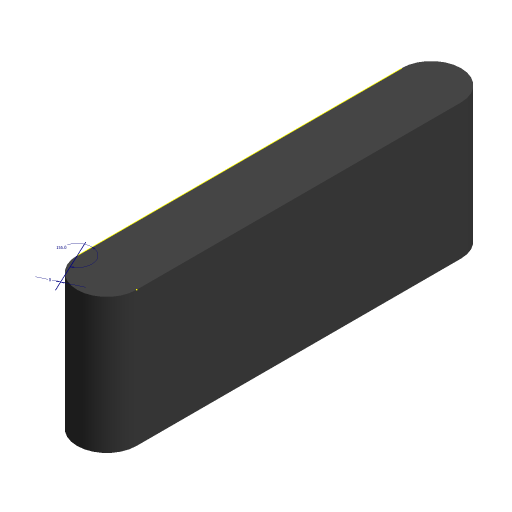
# Autodesk Inventor part: Camera retention
Saved by Autodesk Inventor 2024 (Build 280153000, 153)
## iProperties
Part Number: Camera retention
Material: Generic
Document SubType Name: Modeling
Designer: Jamie
Appearance: Default
Author: Jamie
Autodesk Inventor part; units mm, degrees
ref_plane "YZ Plane" through (0, 0, 0) normal (1, 0, 0) x (0, 1, 0)
ref_plane "XZ Plane" through (0, 0, 0) normal (0, 1, 0) x (-1, 0, 0)
ref_plane "XY Plane" through (0, 0, 0) normal (0, 0, 1) x (1, 0, 0)
sketch "Sketch1" plane through (0, 0, 0) normal (0, 1, 0) x (-1, 0, 0)
  line L0 (0, 0) -> (0, -24)
  arc A0 (4.4, 0) -> (0, 0) centre (2.2, 0) ccw
  arc A1 (0, -24) -> (4.4, -24) centre (2.2, -24) ccw
  line L1 (4.4, 0) -> (4.4, -24)
  dimension "d0" = 24
  constraints: 4 end point, 4 point on circle, 2 centre point, 2 tangent, 1 vertical
  measures "d0" distance of L0.start L0.end
extrude "Extrusion1" add sketch "Sketch1" along normal blind 10
sketch "Sketch2" plane through (0, 10, 0) normal (0, 1, 0) x (1, 0, 0)
  line L0 (-4.9429, 1.1642) -> (-2.9858, -3.0328)
  line L1 (-4.4, 24) -> (-4.4, 0) projected
  point P0 (0, 0)
  dimension "d7" = 25
  dimension "d8" = 0
  constraints: 2 end point
  measures "d7" angle of L1 L0
  measures "d8" distance from line of L1.end L0
body "Solid1"
